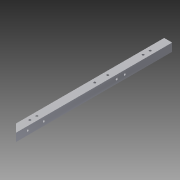
# Autodesk Inventor part: Rebuild Shooter Tower Top Tube 1
Saved by Autodesk Inventor 2014 SP1 (Build 180222100, 222)
## iProperties
Created: 2013-10-25
Part Number: Rebuild Shooter Tower Top Tube 1
Material: Aluminum 6061
Document SubType Name: Modeling
Designer: Moses
Density: 2.71 g/cm^3
Appearance: Aluminum - Flat
Mass: 194.674 g
Surface Area: 915.402 cm^2
Volume: 71.8353 cm^3
Author: Moses
Autodesk Inventor part; units mm, degrees
ref_plane "YZ Plane" through (0, 0, 0) normal (1, 0, 0) x (0, 1, 0)
ref_plane "XZ Plane" through (0, 0, 0) normal (0, 1, 0) x (-1, 0, 0)
ref_plane "XY Plane" through (0, 0, 0) normal (0, 0, 1) x (1, 0, 0)
sketch "Sketch1" plane through (0, 0, 0) normal (0, 0, 1) x (1, 0, 0)
  line L0 (0, 0) -> (25.4, 0)
  line L1 (25.4, 0) -> (25.4, 25.4)
  line L2 (25.4, 25.4) -> (0, 25.4)
  line L3 (0, 25.4) -> (0, 0)
  line L4 (1.5875, 23.8125) -> (23.8125, 23.8125)
  line L5 (23.8125, 23.8125) -> (23.8125, 1.5875)
  line L6 (23.8125, 1.5875) -> (1.5875, 1.5875)
  line L7 (1.5875, 1.5875) -> (1.5875, 23.8125)
  dimension "d0" = 25.4
  dimension "d1" = 25.4
  dimension "d2" = 1.5875
  constraints: 16 end point, 4 parallel, 2 perpendicular, 1 horizontal, 3 other
  measures "d0" distance of L2.end L1.end
  measures "d1" distance of L1.end L0.end
  measures "d2" distance between parallel lines of L1 L5
extrude "Extrusion1" add sketch "Sketch1" along normal blind 495.3
sketch "Sketch2" plane through (0, 25.4, 0) normal (0, 1, 0) x (1, 0, 0)
  line L0 (25.4, 0) -> (0, 0) projected
  line L1 (0, 0) -> (0, -495.3) projected
  line L2 (25.4, -495.3) -> (0, -495.3) projected
  line L3 (12.7, 0) -> (12.7, -495.3) construction
  line L4 (25.4, -495.3) -> (0, -469.9)
  circle A0 centre (12.7, -79.375) radius 3.3782 projected
  circle A1 centre (12.7, -57.15) radius 3.3782 projected
  circle A2 centre (12.7, -438.15) radius 3.3782 projected
  circle A3 centre (12.7, -415.925) radius 3.3782 projected
  circle A4 centre (11.9062, -191.2218) radius 3.3782 projected
  circle A5 centre (11.9062, -232.4968) radius 3.3782 projected
  line L5 (-2.6988, -143.5968) -> (-2.6988, -242.0218) construction
  line L6 (24.6062, -242.0218) -> (-2.6988, -242.0218) construction
  line L7 (24.6062, -143.5968) -> (24.6062, -242.0218) projected
  line L8 (-2.6988, -143.5968) -> (24.6062, -143.5968) construction
  dimension "d6" = 45
  constraints: 4 end point, 2 midpoint, 1 point on line
  measures "d6" angle of L2 L4
extrude "Extrusion2" cut sketch "Sketch2" against normal blind 25.4
sketch "Sketch3" plane through (25.4, 0, 0) normal (1, 0, 0) x (0, 0, -1)
  circle A0 centre (-149.9468, 12.7434) radius 3.3782 projected
  circle A1 centre (-175.3468, 12.7434) radius 3.3782 projected
  circle A2 centre (-406.4, 12.7) radius 3.3782 projected
  circle A3 centre (-457.2, 12.7) radius 3.3782 projected
extrude "Extrusion3" cut sketch "Sketch3" against normal blind 25.4
body "Solid1"
